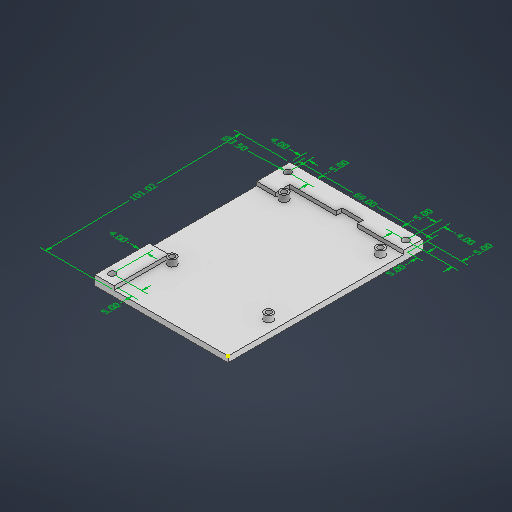
# Autodesk Inventor part: ThridPrototypeRaspPiBed
Saved by Autodesk Inventor 2026 (Build 300175000, 175)
## iProperties
Created: 2025-07-05
Part Number: ThridPrototypeRaspPiBed
Material: Generic
Document SubType Name: Modeling
Designer: jsmal
Density: 1 g/cm^3
Appearance: Default
Author: jsmal
Autodesk Inventor part; units mm, degrees
ref_plane "YZ Plane" through (0, 0, 0) normal (1, 0, 0) x (0, 1, 0)
ref_plane "XZ Plane" through (0, 0, 0) normal (0, 1, 0) x (-1, 0, 0)
ref_plane "XY Plane" through (0, 0, 0) normal (0, 0, 1) x (1, 0, 0)
sketch "Sketch1" plane through (0, 0, 0) normal (0, 1, 0) x (-1, 0, 0)
  line L0 (0, 0) -> (59, 0)
  line L1 (59, 0) -> (59, -91)
  line L2 (59, -91) -> (0, -91)
  line L3 (0, -91) -> (0, 0)
  dimension "d0" = 59
  dimension "d1" = 91
  constraints: 8 end point, 2 parallel, 1 horizontal, 1 perpendicular
  measures "d0" distance of L1.end L2.end
  measures "d1" distance of L0.end L1.end
extrude "Extrusion1" add sketch "Sketch1" along normal blind 3
sketch "Sketch2" plane through (0, 3, 0) normal (0, 1, 0) x (1, 0, 0)
  line L0 (0, 0) -> (-69, 0)
  line L1 (-69, 0) -> (-69, 101)
  line L2 (-69, 101) -> (0, 101)
  line L3 (0, 101) -> (0, 0)
  line L4 (-59, 91) -> (-59, 0) projected
  line L5 (0, 91) -> (-59, 91) projected
  dimension "d4" = 10
  dimension "d5" = 10
  constraints: 8 end point, 2 parallel, 1 horizontal, 1 perpendicular
  measures "d4" distance between parallel lines of L4 L1
  measures "d5" distance between parallel lines of L2 L5
extrude "Extrusion2" add sketch "Sketch2" along normal blind 2 and the other way blind 3 contours L0 L1 L2 L3 L5 L4
sketch "Sketch3" plane through (0, 3, 0) normal (0, 1, 0) x (1, 0, 0)
  circle A0 centre (-56, 27) radius 1.35
  line L0 (-59, 0) -> (-59, 91) projected
  line L1 (-59, 0) -> (0, 0) projected
  circle A1 centre (-6, 27) radius 1.35
  line L2 (0, 0) -> (0, 91) projected
  circle A2 centre (-56, 85) radius 1.35
  line L3 (-59, 91) -> (0, 91) projected
  circle A3 centre (-6, 85) radius 1.35
  dimension "d10" = 2.7
  dimension "d11" = 3
  dimension "d12" = 27
  dimension "d13" = 2.7
  dimension "d14" = 6
  dimension "d15" = 27
  dimension "d16" = 2.7
  dimension "d17" = 3
  dimension "d18" = 6
  dimension "d19" = 2.7
  dimension "d20" = 6
  dimension "d21" = 6
  constraints: 4 centre point
  measures "d10" diameter of A0
  measures "d11" distance from line of L0 A0.centre
  measures "d12" distance from line of L1 A0.centre
  measures "d13" diameter of A1
  measures "d14" distance from line of L2 A1.centre
  measures "d15" distance from line of L1 A1.centre
  measures "d16" diameter of A2
  measures "d17" distance from line of L0 A2.centre
  measures "d18" distance from line of L3 A2.centre
  measures "d19" diameter of A3
  measures "d20" distance from line of L2 A3.centre
  measures "d21" distance from line of L3 A3.centre
extrude "Extrusion3" cut sketch "Sketch3" against normal blind 3 contours A0 | A1 | A2 | A3
sketch "Sketch4" plane through (0, 3, 0) normal (0, 1, 0) x (1, 0, 0)
  point P0 (0, 0)
sketch "Sketch5" plane through (0, 3, 0) normal (0, 1, 0) x (1, 0, 0)
  circle A0 centre (-56, 27) radius 2.25
  circle A1 centre (-56, 27) radius 1.35 projected
  circle A2 centre (-56, 85) radius 2.25
  circle A3 centre (-6, 85) radius 2.25
  circle A4 centre (-6, 85) radius 1.35 projected
  circle A5 centre (-56, 85) radius 1.35 projected
  circle A6 centre (-6, 27) radius 2.25
  circle A7 centre (-6, 27) radius 1.35 projected
  point P0 (0, 0)
  dimension "d24" = 0
  dimension "d25" = 0
  dimension "d26" = 4.5
  dimension "d27" = 4.5
  dimension "d28" = 4.5
  dimension "d29" = 0
  dimension "d30" = 0
  dimension "d31" = 0
  dimension "d32" = 4.5
  dimension "d33" = 0.9
  dimension "d34" = 0.9
  dimension "d35" = 0.9
  dimension "d36" = 0.9
  constraints: 4 centre point
  measures "d24" distance of A1.centre A0.centre
  measures "d25" distance of A1.centre A0.centre
  measures "d26" diameter of A0
  measures "d27" diameter of A2
  measures "d28" diameter of A3
  measures "d29" distance of A3.centre A4.centre
  measures "d30" distance of A4.centre A3.centre
  measures "d31" distance of A5.centre A2.centre
  measures "d32" diameter of A6
  measures "d33" radial gap between concentric circles of A6 A7
  measures "d34" radial gap between concentric circles of A1 A0
  measures "d35" radial gap between concentric circles of A5 A2
  measures "d36" radial gap between concentric circles of A4 A3
extrude "Extrusion4" add sketch "Sketch5" along normal blind 3.2
sketch "Sketch6" plane through (-59, 3, -91) normal (0, 0, 1) x (1, 0, 0)
  line L0 (0, 2) -> (59, 2) projected
  line L1 (0, 0) -> (59, 0) projected
  line L2 (24, 2) -> (35, 2)
  line L3 (35, 2) -> (35, 0)
  line L4 (35, 0) -> (24, 0)
  line L5 (24, 0) -> (24, 2)
  line L6 (59, 0) -> (59, 2) projected
  line L7 (0, 0) -> (0, 2) projected
  point P0 (59, -3)
  point P1 (24, 0)
  dimension "d39" = 11
  dimension "d40" = 24
  dimension "d41" = 24
  constraints: 8 end point, 2 parallel, 2 point on line, 1 horizontal, 1 perpendicular
  measures "d39" distance of L3.end L4.end
  measures "d40" distance between parallel lines of L6 L3
  measures "d41" distance between parallel lines of L7 L5
extrude "Extrusion5" cut sketch "Sketch6" against normal blind 3 contours L0 L3 L1 L5
sketch "Sketch7" plane through (0, 5, 0) normal (0, 1, 0) x (1, 0, 0)
  circle A0 centre (-65, 5) radius 1.75
  line L0 (-69, 101) -> (-69, 0) projected
  line L1 (-69, 0) -> (-59, 0) projected
  circle A1 centre (-65, 96) radius 1.75
  line L2 (0, 101) -> (-69, 101) projected
  circle A2 centre (-4, 96) radius 1.75
  line L3 (0, 91) -> (0, 101) projected
  point P0 (0, 0)
  dimension "d44" = 3.5
  dimension "d45" = 4
  dimension "d46" = 5
  dimension "d47" = 3.5
  dimension "d48" = 4
  dimension "d49" = 5
  dimension "d50" = 3.5
  dimension "d51" = 5
  dimension "d52" = 4
  constraints: 3 centre point
  measures "d44" diameter of A0
  measures "d45" distance from line of L0 A0.centre
  measures "d46" distance from line of L1 A0.centre
  measures "d47" diameter of A1
  measures "d48" distance from line of L0 A1.centre
  measures "d49" distance from line of L2 A1.centre
  measures "d50" diameter of A2
  measures "d51" distance from line of L2 A2.centre
  measures "d52" distance from line of L3 A2.centre
extrude "Extrusion6" cut sketch "Sketch7" against normal blind 19
sketch "Sketch8" plane through (0, 5, 0) normal (0, 1, 0) x (1, 0, 0)
  line L0 (-69, 101) -> (-69, 0) projected
  line L1 (-59, 83.8) -> (-69, 83.8)
  line L2 (-69, 83.8) -> (-69, 28.2)
  line L3 (-69, 28.2) -> (-59, 28.2)
  line L4 (-59, 28.2) -> (-59, 83.8)
  line L5 (-59, 0) -> (-59, 91) projected
  circle A0 centre (-56, 27) radius 2.25 projected
  circle A1 centre (-56, 85) radius 1.35 projected
  point P0 (0, 0)
  dimension "d55" = 0
  dimension "d56" = 1.2
  dimension "d57" = 1.2
  constraints: 8 end point, 2 parallel, 1 horizontal, 1 perpendicular, 1 point on line
  measures "d55" distance between parallel lines of L5 L4
  measures "d56" distance from line of A0.centre L3
  measures "d57" distance from line of A1.centre L1
extrude "Extrusion7" cut sketch "Sketch8" against normal blind 2 contours L1 L4 L3 L0
body "Solid1"
